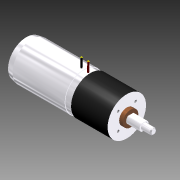
# Autodesk Inventor part: 409A587
Saved by Autodesk Inventor 2011 (Build 150239000, 239)
## iProperties
Category: Motors
Shininess: 64.0
Length Units: 11269
Angle Units: 11279
Time Units: 11290
Mass Units: 11283
Length Display Precision: 3
Angle Display Precision: 2
Compacted: True
Part Number: 409A587
Document SubType Name: Modeling
Created: 2005-01-08
Manufacturer: Standard
Standards Organization: Custom
Description: Globe Motor with Drive Assembly
Project: FIRST
Catalog Web Link: http://www.globe-motors.com/home.html
Vendor: Globe Motors
Density: 1 g/cm^3
Density: 0.0
Volumn: 0.0
Area: 0.0
PropertySet Name: Model Information
Control State: 0
Master: False
Checked Out: False
Title: Motor - Globe
Author: Autodesk, Inc.
Autodesk Inventor part; units mm, degrees
ref_plane "YZ Plane" through (0, 0, 0) normal (1, 0, 0) x (0, 1, 0)
sketch "Sketch1" plane through (0, 0, 0) normal (0, 0, 1) x (1, 0, 0)
  circle A0 centre (0, 0) radius 20
  dimension "d0" = 40
  constraints: 1 centre point, 1 coincident
  measures "d0" diameter of A0
extrude "Extrusion1" add sketch "Sketch1" along normal blind 60
sketch "Sketch2" plane through (0, 0, 60) normal (0, 0, 1) x (1, 0, 0)
  circle A0 centre (0, 0) radius 20 projected
  circle A1 centre (0, 0) radius 19.345
  constraints: 1 centre point, 1 coincident
extrude "Extrusion2" add sketch "Sketch2" along normal blind 6.6 contours A1
sketch "Sketch3" plane through (0, 0, 66.6) normal (0, 0, 1) x (1, 0, 0)
  circle A0 centre (0, 0) radius 19.345 projected
  circle A1 centre (0, 0) radius 20
  dimension "d5" = 40
  constraints: 1 centre point, 1 coincident
  measures "d5" diameter of A1
extrude "Extrusion3" add sketch "Sketch3" along normal blind 38 contours A0 | A1
sketch "Sketch4" plane through (0, 0, 104.6) normal (0, 0, 1) x (1, 0, 0)
  circle A0 centre (0, 0) radius 20 projected
  circle A1 centre (0, 0) radius 8
  dimension "d8" = 16
  constraints: 1 centre point, 1 coincident
  measures "d8" diameter of A1
extrude "Extrusion4" add sketch "Sketch4" along normal blind 4 contours A1
sketch "Sketch5" plane through (0, 0, 108.6) normal (0, 0, 1) x (1, 0, 0)
  circle A0 centre (0, 0) radius 8 projected
  line L0 (3.75, 2.9155) -> (3.75, -2.9155)
  line L1 (-3.75, -2.9155) -> (-3.75, 2.9155)
  arc A1 (-3.75, -2.9155) -> (3.75, -2.9155) centre (0, 0) ccw
  arc A2 (3.75, 2.9155) -> (-3.75, 2.9155) centre (0, 0) ccw
  point P0 (-3.75, 0)
  point P1 (0, 5.9024)
  dimension "d13" = 4.75
  dimension "d14" = 4.75
  dimension "d15" = 7.5
  dimension "d16" = 3.75
  dimension "d17" = 7.5
  dimension "d18" = 5.9024
  constraints: 4 end point, 4 point on circle, 2 centre point, 1 coincident, 1 horizontal alignment, 1 parallel, 1 vertical, 1 vertical alignment
  measures "d13" radius of A2
  measures "d14" radius of A1
  measures "d15" distance between parallel lines of L0 L1
  measures "d16" distance from line of A0.centre L0
  measures "d17" distance from line of point (-3.75, 0) L0
  measures "d18" distance of point (0, 5.902) A0.centre
extrude "Extrusion5" add sketch "Sketch5" along normal blind 14 contours L0 A1 L1 A2
sketch "Sketch6" plane through (0, 0, 122.6) normal (0, 0, 1) x (1, 0, 0)
  line L0 (3.75, 2.9155) -> (3.75, -2.9155) projected
  arc A0 (3.75, 2.9155) -> (-3.75, 2.9155) centre (0, 0) ccw projected
  line L1 (-3.75, -2.9155) -> (-3.75, 2.9155) projected
  arc A1 (-3.75, -2.9155) -> (3.75, -2.9155) centre (0, 0) ccw projected
  circle A2 centre (0, 0) radius 3.25
  dimension "d21" = 6.5
  constraints: 1 centre point, 1 coincident
  measures "d21" diameter of A2
extrude "Extrusion6" add sketch "Sketch6" along normal blind 10 contours A2
chamfer "Chamfer1" distance 1 angle 45 1 edges at (-3.25, 0, 132.6)
chamfer "Chamfer2" distance 1 angle 80 1 edges at (-20, 0, 0) measured on face at (-2.364, 6.2334, 0)
ref_plane "Work Plane1" through (-19.345, 0, 60) normal (1, 0, 0) x (0, 1, 0)
ref_plane "Work Plane2" through (-19.095, 0, 60) normal (1, 0, 0) x (0, 1, 0)
sketch "Sketch8" plane through (-19.095, 0, 60) normal (1, 0, 0) x (0, 1, 0)
  circle A0 centre (0.0498, -2.6078) radius 0.75
  circle A1 centre (0, 4.3902) radius 0.75
  dimension "d31" = 1.5
  dimension "d32" = 1.5
  constraints: 2 centre point
  measures "d31" diameter of A1
  measures "d32" diameter of A0
extrude "Extrusion7" add sketch "Sketch8" against normal blind 10
sketch "Sketch9" plane through (0, 0, 104.6) normal (0, 0, 1) x (1, 0, 0)
  circle A0 centre (0, 0) radius 8 projected
  circle A1 centre (0, 0) radius 20 projected
  line L0 (-9, 9) -> (9, 9)
  line L1 (9, 9) -> (9, -9)
  line L2 (9, -9) -> (-9, -9)
  line L3 (-9, -9) -> (-9, 9)
  point P0 (0, 9)
  point P1 (-9, 0)
  dimension "d35" = 18
  dimension "d36" = 18
  constraints: 8 end point, 2 midpoint, 2 parallel, 1 horizontal, 1 horizontal alignment, 1 perpendicular, 1 vertical alignment
  measures "d35" distance of L0.start L0.end
  measures "d36" distance of L0.end L1.end
hole "Hole1" at (-9, 9, 104.6) at (9, 9, 104.6) at (9, -9, 104.6) at (-9, -9, 104.6) direction (0, 0, -1) diameter 2.487 depth 8 tip angle 118 thread size "5-40 UNC" class "2B" standard "ANSI Unified Screw Threads"
equation "\"d32\" = d31"
equation "\"d36\" = d35"
body "Solid1"
